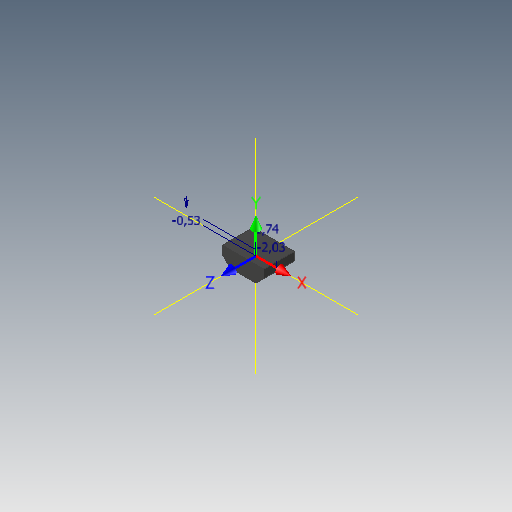
# Autodesk Inventor part: HallEffectSensor
Saved by Autodesk Inventor 2021.4 (Build 254397000, 397)
## iProperties
Created: 2022-09-12
Part Number: HallEffectSensor
Material: Generisch
Document SubType Name: Modeling
Designer: alexw
Density: 1 g/cm^3
Appearance: Vorgabe
Mass: 0.0173442 g
Surface Area: 0.42637 cm^2
Volume: 0.0173442 cm^3
Author: alexw
Autodesk Inventor part; units mm, degrees
ref_plane "YZ Plane" through (0, 0, 0) normal (1, 0, 0) x (0, 1, 0)
ref_plane "XZ Plane" through (0, 0, 0) normal (0, 1, 0) x (-1, 0, 0)
ref_plane "XY Plane" through (0, 0, 0) normal (0, 0, 1) x (1, 0, 0)
sketch "Sketch1" plane through (0, 0, 0) normal (0, 0, 1) x (1, 0, 0)
  line L0 (-2.03, 0.81) -> (2.03, 0.81)
  line L1 (2.03, 0.81) -> (2.03, 0)
  line L2 (2.03, 0) -> (1.25, -0.76)
  line L3 (1.25, -0.76) -> (-1.25, -0.76)
  line L4 (-1.25, -0.76) -> (-2.03, 0)
  line L5 (-2.03, 0) -> (-2.03, 0.81)
  line L6 (-2.03, 0) -> (2.03, 0) construction
  line L7 (0, 0.81) -> (0, -0.76) construction
  point P0 (0, 0)
  point P1 (0, 0)
  dimension "d0" = 4.06
  dimension "d1" = 2.5
  dimension "d2" = 1.57
  dimension "d3" = 0.76
  constraints: 16 end point, 3 midpoint, 2 horizontal, 2 parallel, 1 coincident, 1 equal length, 1 perpendicular
  measures "d0" distance between parallel lines of L1 L5
  measures "d1" distance of L2.end L3.end
  measures "d2" distance between parallel lines of L0 L3
  measures "d3" distance between parallel lines of L6 L3
extrude "Extrusion1" add sketch "Sketch1" along normal blind 3
sketch3d "3D Sketch1"
body "Solid1"
